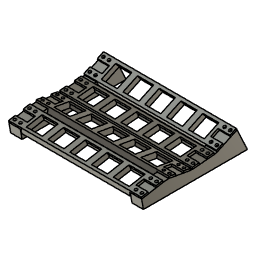
generator (Autodesk Fusion 360 design; units mm, degrees)
Autodesk Fusion 360 part; units mm, degrees
sketch "sketchRails" plane through (0, 0, 0) normal (1, 0, 0) x (0, 1, 0)
  line L0 (-1.7973, 10.1928) -> (16.9633, 13.5008)
  line L1 (22.5, 13.9365) -> (41.2606, 10.6285)
  line L2 (42.9622, 10.5542) -> (61.9397, 12.2146)
  line L3 (64.1312, 12.8018) -> (81.3964, 20.8527)
  line L4 (0, 0) -> (87.5485, 7.6595) construction
  line L5 (42.7693, 17.0622) -> (60.9996, 18.6571) construction
  line L6 (61.7241, 18.8513) -> (78.3095, 26.5852) construction
  line L7 (42.02, 17.0949) -> (23.998, 20.2727) construction
  line L8 (15.4653, 19.8369) -> (-2.5567, 16.6591) construction
  line L9 (78.3095, 26.5852) -> (72.1582, 32.3231) construction
  line L10 (72.1582, 32.3231) -> (61.2825, 27.2517) construction
  line L11 (61.2825, 27.2517) -> (61.7241, 18.8513) construction
  line L12 (60.9996, 18.6571) -> (57.1818, 26.1529) construction
  line L13 (57.1818, 26.1529) -> (45.2275, 25.1071) construction
  line L14 (45.2275, 25.1071) -> (42.7693, 17.0622) construction
  line L15 (42.02, 17.0949) -> (40.2723, 25.3234) construction
  line L16 (40.2723, 25.3234) -> (28.4546, 27.4072) construction
  line L17 (28.4546, 27.4072) -> (23.998, 20.2727) construction
  line L18 (15.4653, 19.8369) -> (11.0087, 26.9714) construction
  line L19 (11.0087, 26.9714) -> (-0.809, 24.8876) construction
  line L20 (-0.809, 24.8876) -> (-2.5567, 16.6591) construction
  line L21 (7.583, 11.8468) -> (6.4543, 18.248) construction
  line L22 (31.8803, 12.2825) -> (33.009, 18.6838) construction
  line L23 (52.451, 11.3844) -> (51.8844, 17.8597) construction
  line L24 (72.7638, 16.8272) -> (70.0168, 22.7182) construction
  line L25 (-1.7973, 10.1928) -> (16.9633, 13.5008)
  line L26 (16.9633, 13.5008) -> (17.2412, 11.9251)
  line L27 (17.2412, 11.9251) -> (-1.5194, 8.6171)
  line L28 (-1.5194, 8.6171) -> (-1.7973, 10.1928)
  line L29 (22.5, 13.9365) -> (41.2606, 10.6285)
  line L30 (41.2606, 10.6285) -> (40.9827, 9.0528)
  line L31 (40.9827, 9.0528) -> (22.2221, 12.3608)
  line L32 (22.2221, 12.3608) -> (22.5, 13.9365)
  line L33 (42.9622, 10.5542) -> (61.9397, 12.2146)
  line L34 (61.9397, 12.2146) -> (62.0792, 10.6206)
  line L35 (62.0792, 10.6206) -> (43.1016, 8.9603)
  line L36 (43.1016, 8.9603) -> (42.9622, 10.5542)
  line L37 (64.1312, 12.8018) -> (81.3964, 20.8527)
  line L38 (81.3964, 20.8527) -> (82.0726, 19.4026)
  line L39 (82.0726, 19.4026) -> (64.8074, 11.3517)
  line L40 (64.8074, 11.3517) -> (64.1312, 12.8018)
  line L41 (43.1016, 8.9603) -> (40.9827, 9.0528)
  line L42 (22.2221, 12.3608) -> (17.2412, 11.9251)
  line L43 (-1.5194, 8.6171) -> (0, 0)
  line L44 (42.7693, 17.0622) -> (42.02, 17.0949)
  line L45 (61.7241, 18.8513) -> (60.9996, 18.6571)
  line L46 (62.0792, 10.6206) -> (64.8074, 11.3517)
  line L47 (61.3618, 18.7542) -> (63.4433, 10.9862) construction
  line L48 (42.3946, 17.0786) -> (42.0422, 9.0066) construction
  line L49 (0, 0) -> (91.1201, 0)
  line L50 (91.1201, 0) -> (82.0726, 19.4026)
  dimension "d1" = 19.05
  dimension "d2" = 19.05
  dimension "d3" = 19.05
  dimension "d4" = 19.05
  dimension "d6" = 5
  dimension "d7" = 15
  dimension "d8" = 20
  dimension "d9" = 18.3
  dimension "d10" = 18.3
  dimension "d11" = 18.3
  dimension "d12" = 18.3
  dimension "d13" = 12
  dimension "d14" = 12
  dimension "d15" = 12
  dimension "d16" = 12
  dimension "d17" = 7.8
  dimension "d18" = 7.8
  dimension "d19" = 7.8
  dimension "d20" = 7.8
  dimension "d21" = 6.5
  dimension "d22" = 6.5
  dimension "d23" = 6.5
  dimension "d24" = 6.5
  dimension "d25" = 1.6
  dimension "d26" = 1.6
  dimension "d27" = 1.6
  dimension "d28" = 1.6
  dimension "d30" = 0.75
  dimension "d31" = 0.75
  dimension "d32" = 5
  dimension "d34" = 5
  dimension "d40" = 8.75
  dimension "validationClearance" = 8.9603
  constraint parallel L2 L4
  constraint parallel L2 L5
  constraint parallel L1 L7
  constraint parallel L0 L8
  constraint parallel L3 L6
  constraint parallel L6 L10
  constraint parallel L5 L13
  constraint parallel L7 L16
  constraint parallel L8 L19
  constraint equal L18 L20
  constraint equal L15 L17
  constraint equal L12 L14
  constraint equal L9 L11
  constraint midpoint L0 L21.start
  constraint midpoint L8 L21.end
  constraint midpoint L1 L22.start
  constraint midpoint L7 L22.end
  constraint midpoint L2 L23.start
  constraint midpoint L5 L23.end
  constraint midpoint L3 L24.start
  constraint midpoint L6 L24.end
  constraint perpendicular L3 L24
  constraint perpendicular L2 L23
  constraint perpendicular L1 L22
  constraint perpendicular L0 L21
  constraint perpendicular L25 L26
  constraint parallel L25 L27
  constraint parallel L26 L28
  constraint perpendicular L29 L30
  constraint parallel L29 L31
  constraint parallel L30 L32
  constraint perpendicular L33 L34
  constraint parallel L33 L35
  constraint parallel L34 L36
  constraint perpendicular L37 L38
  constraint parallel L37 L39
  constraint parallel L38 L40
  constraint coincident L4 L43.end
  constraint perpendicular L27 L43
  constraint midpoint L45 L47.start
  constraint midpoint L46 L47.end
  constraint midpoint L44 L48.start
  constraint midpoint L41 L48.end
  constraint perpendicular L41 L48
  constraint perpendicular L45 L47
  constraint perpendicular L44 L48
  constraint parallel L4 L42
  constraint horizontal L49
  constraint perpendicular L39 L50
  constraint coincident L4.start L43.end
  constraint coincident L4.end L50
  measures "d1" distance of L0.start L0.end
  measures "d2" distance of L1.start L1.end
  measures "d3" distance of L2.start L2.end
  measures "d4" distance of L3.start L3.end
  measures "d6" angle of L0 L4
  measures "d7" angle of L1 L4
  measures "d8" angle of L3 L4
  measures "d9" distance of L5.start L5.end
  measures "d10" distance of L6.start L6.end
  measures "d11" distance of L7.start L7.end
  measures "d12" distance of L8.start L8.end
  measures "d13" distance of L15.end L16.end
  measures "d14" distance of L18.end L19.end
  measures "d15" distance of L12.end L13.end
  measures "d16" distance of L9.end L10.end
  measures "d17" distance of L5 L13
  measures "d18" distance of L6 L10
  measures "d19" distance of L7 L16
  measures "d20" distance of L8 L19
  measures "d21" distance of L0 L8
  measures "d22" distance of L1 L7
  measures "d23" distance of L2 L5
  measures "d24" distance of L3 L6
  measures "d25" distance of L0.start L27.end
  measures "d26" distance of L1.start L31.end
  measures "d27" distance of L2.start L35.end
  measures "d28" distance of L3.start L39.end
  measures "d30" distance of L5.start L7.start
  measures "d31" distance of L5.end L6.start
  measures "d32" distance of L26.end L31.end
  measures "d34" angle of L4 L49
  measures "d40" distance of L27.end L4.start
  measures "validationClearance" distance of L35.end L49
extrude "extrudeRailLeft" add sketch "sketchRails" along normal blind 10 contours L27 L31 L35 L39 L41 L42 L43 L46 L49 L50 makes body 1
extrude "extrudeRailRight" add sketch "sketchRails" along normal blind 10 from surface at 106.3 separate body contours L27 L31 L35 L39 L41 L42 L43 L46 L49 L50 makes body 2
sketch "sketchPlateTop" plane through (0, 7.2271, -15.4985) normal (0, -0.422618, 0.906308) x (1, 0, 0)
  line L0 (0, 82.5829) -> (0, 63.5329)
  line L1 (0, 63.5329) -> (10, 63.5329)
  line L2 (10, 63.5329) -> (10, 82.5829)
  line L3 (10, 82.5829) -> (0, 82.5829)
  line L4 (106.3, 82.5829) -> (106.3, 63.5329)
  line L5 (106.3, 63.5329) -> (116.3, 63.5329)
  line L6 (116.3, 63.5329) -> (116.3, 82.5829)
  line L7 (116.3, 82.5829) -> (106.3, 82.5829)
  line L8 (0, 82.5829) -> (116.3, 82.5829)
  line L9 (116.3, 82.5829) -> (116.3, 63.5329)
  line L10 (116.3, 63.5329) -> (0, 63.5329)
  line L11 (0, 63.5329) -> (0, 82.5829)
  line L12 (0, 76.5829) -> (10.525, 76.5829)
  line L13 (10.525, 76.5829) -> (10.525, 69.5329)
  line L14 (10.525, 69.5329) -> (0, 69.5329)
  line L15 (0, 69.5329) -> (0, 76.5829)
  line L16 (116.3, 69.5329) -> (105.775, 69.5329)
  line L17 (105.775, 69.5329) -> (105.775, 76.5829)
  line L18 (105.775, 76.5829) -> (116.3, 76.5829)
  line L19 (116.3, 76.5829) -> (116.3, 69.5329)
  line L20 (13.05, 80.0579) -> (27.05, 80.0579)
  line L21 (27.05, 80.0579) -> (27.05, 66.0579)
  line L22 (27.05, 66.0579) -> (13.05, 66.0579)
  line L23 (13.05, 66.0579) -> (13.05, 80.0579)
  line L24 (32.1, 80.0579) -> (46.1, 80.0579)
  line L25 (46.1, 80.0579) -> (46.1, 66.0579)
  line L26 (46.1, 66.0579) -> (32.1, 66.0579)
  line L27 (32.1, 66.0579) -> (32.1, 80.0579)
  line L28 (51.15, 80.0579) -> (65.15, 80.0579)
  line L29 (65.15, 80.0579) -> (65.15, 66.0579)
  line L30 (65.15, 66.0579) -> (51.15, 66.0579)
  line L31 (51.15, 66.0579) -> (51.15, 80.0579)
  line L32 (70.2, 80.0579) -> (84.2, 80.0579)
  line L33 (84.2, 80.0579) -> (84.2, 66.0579)
  line L34 (84.2, 66.0579) -> (70.2, 66.0579)
  line L35 (70.2, 66.0579) -> (70.2, 80.0579)
  line L36 (89.25, 80.0579) -> (103.25, 80.0579)
  line L37 (103.25, 80.0579) -> (103.25, 66.0579)
  line L38 (103.25, 66.0579) -> (89.25, 66.0579)
  line L39 (89.25, 66.0579) -> (89.25, 80.0579)
  line L40 (5, 63.5329) -> (5, 69.5329) construction
  line L41 (5, 66.5329) -> (10, 66.5329) construction
  line L42 (5, 66.5329) -> (0, 66.5329) construction
  circle A0 centre (2.5, 66.5329) radius 1.5 construction
  circle A1 centre (7.5, 66.5329) radius 1.5 construction
  circle A2 centre (2.5, 66.5329) radius 1.2
  circle A3 centre (7.5, 66.5329) radius 1.2
  line L43 (0, 73.0579) -> (116.3, 73.0579) construction
  line L44 (58.15, 82.5829) -> (58.15, 63.5329) construction
  circle A4 centre (2.5, 79.5829) radius 1.2
  circle A5 centre (7.5, 79.5829) radius 1.2
  circle A6 centre (108.8, 79.5829) radius 1.2
  circle A7 centre (113.8, 79.5829) radius 1.2
  circle A8 centre (113.8, 66.5329) radius 1.2
  circle A9 centre (108.8, 66.5329) radius 1.2
  dimension "d47" = 10.525
  dimension "d48" = 7.05
  dimension "d49" = 10.525
  dimension "d50" = 7.05
  dimension "d51" = 6
  dimension "d52" = 6
  dimension "d53" = 14
  dimension "d54" = 14
  dimension "d55" = 2.525
  dimension "d56" = 2.525
  dimension "d59" = 19.05
  dimension "d60" = 0
  dimension "d138" = 3
  dimension "d139" = 3
  dimension "d140" = 2.4
  dimension "d141" = 2.4
  constraint horizontal L8
  constraint vertical L9
  constraint horizontal L10
  constraint vertical L11
  constraint coincident L5.end L6.start
  constraint coincident L0.start L3.end
  constraint horizontal L12
  constraint vertical L13
  constraint horizontal L14
  constraint vertical L15
  constraint coincident L0 L12.start
  constraint horizontal L16
  constraint vertical L17
  constraint horizontal L18
  constraint vertical L19
  constraint coincident L6 L16.start
  constraint horizontal L20
  constraint vertical L21
  constraint horizontal L22
  constraint vertical L23
  constraint midpoint L1 L40.start
  constraint coincident L14 L40.end
  constraint perpendicular L14 L40
  constraint midpoint L40 L41.start
  constraint coincident L2 L41.end
  constraint perpendicular L2 L41
  constraint coincident L11 L42.end
  constraint perpendicular L11 L42
  constraint midpoint L42 A0.centre
  constraint midpoint L41 A1.centre
  constraint concentric A0 A2
  constraint concentric A1 A3
  constraint midpoint L15 L43.start
  constraint midpoint L19 L43.end
  constraint midpoint L8 L44.start
  constraint midpoint L10 L44.end
  constraint symmetric A2 L43 A4
  constraint symmetric A3 L43 A5
  constraint symmetric A2 L44 A8
  constraint symmetric A3 L44 A9
  constraint symmetric L44 A4 A7
  constraint symmetric L44 A5 A6
  measures "d47" distance of L12.start L12.end
  measures "d48" distance of L12.start L14.end
  measures "d49" distance of L16.start L16.end
  measures "d50" distance of L16.start L18.end
  measures "d51" distance of L8 L12
  measures "d52" distance of L8 L18
  measures "d53" distance of L20.start L20.end
  measures "d54" distance of L20.start L22.end
  measures "d55" distance of L13 L23
  measures "d56" distance of L8 L20
  measures "d138" diameter of A0
  measures "d139" diameter of A1
  measures "d140" diameter of A2
  measures "d141" diameter of A3
hole "holeRailsTop" at (2.5, 79.3537, 18.1347) at (7.5, 79.3537, 18.1347) at (7.5, 67.5263, 12.6195) at (2.5, 67.5263, 12.6195) at (108.8, 79.3537, 18.1347) at (113.8, 79.3537, 18.1347) at (113.8, 67.5263, 12.6195) at (108.8, 67.5263, 12.6195) direction (0, 0.422618, -0.906308) diameter 1.8 depth 5 tip angle 180 bodies 1 2
extrude "extrudePlateTop" add sketch "sketchPlateTop" along normal blind 1.6 separate body contours L0 L2 L3 L8 L11 L12 | L2 L4 L8 L10 L12 L13 L14 L16 L17 L18 | L0 L1 L2 L10 L11 L14 | L4 L6 L7 L8 L9 L18 | L4 L5 L6 L9 L10 L16 makes body 3
sketch "sketchPlateMiddle" plane through (0, -0.4506, 5.15) normal (0, -0.087156, 0.996195) x (1, 0, 0)
  line L0 (0, 62.7686) -> (0, 43.7186)
  line L1 (0, 43.7186) -> (10, 43.7186)
  line L2 (10, 43.7186) -> (10, 62.7686)
  line L3 (10, 62.7686) -> (0, 62.7686)
  line L4 (106.3, 62.7686) -> (106.3, 43.7186)
  line L5 (106.3, 43.7186) -> (116.3, 43.7186)
  line L6 (116.3, 43.7186) -> (116.3, 62.7686)
  line L7 (116.3, 62.7686) -> (106.3, 62.7686)
  line L8 (0, 62.7686) -> (116.3, 62.7686)
  line L9 (116.3, 62.7686) -> (116.3, 43.7186)
  line L10 (116.3, 43.7186) -> (0, 43.7186)
  line L11 (0, 43.7186) -> (0, 62.7686)
  line L12 (0, 56.7686) -> (10.525, 56.7686)
  line L13 (10.525, 56.7686) -> (10.525, 49.7186)
  line L14 (10.525, 49.7186) -> (0, 49.7186)
  line L15 (0, 49.7186) -> (0, 56.7686)
  line L16 (116.3, 49.7186) -> (105.775, 49.7186)
  line L17 (105.775, 49.7186) -> (105.775, 56.7686)
  line L18 (105.775, 56.7686) -> (116.3, 56.7686)
  line L19 (116.3, 56.7686) -> (116.3, 49.7186)
  line L20 (13.05, 60.2436) -> (27.05, 60.2436)
  line L21 (27.05, 60.2436) -> (27.05, 46.2436)
  line L22 (27.05, 46.2436) -> (13.05, 46.2436)
  line L23 (13.05, 46.2436) -> (13.05, 60.2436)
  line L24 (32.1, 60.2436) -> (46.1, 60.2436)
  line L25 (46.1, 60.2436) -> (46.1, 46.2436)
  line L26 (46.1, 46.2436) -> (32.1, 46.2436)
  line L27 (32.1, 46.2436) -> (32.1, 60.2436)
  line L28 (51.15, 60.2436) -> (65.15, 60.2436)
  line L29 (65.15, 60.2436) -> (65.15, 46.2436)
  line L30 (65.15, 46.2436) -> (51.15, 46.2436)
  line L31 (51.15, 46.2436) -> (51.15, 60.2436)
  line L32 (70.2, 60.2436) -> (84.2, 60.2436)
  line L33 (84.2, 60.2436) -> (84.2, 46.2436)
  line L34 (84.2, 46.2436) -> (70.2, 46.2436)
  line L35 (70.2, 46.2436) -> (70.2, 60.2436)
  line L36 (89.25, 60.2436) -> (103.25, 60.2436)
  line L37 (103.25, 60.2436) -> (103.25, 46.2436)
  line L38 (103.25, 46.2436) -> (89.25, 46.2436)
  line L39 (89.25, 46.2436) -> (89.25, 60.2436)
  line L40 (5, 43.7186) -> (5, 49.7186) construction
  line L41 (5, 46.7186) -> (0, 46.7186) construction
  line L42 (5, 46.7186) -> (10, 46.7186) construction
  circle A0 centre (2.5, 46.7186) radius 1.2
  circle A1 centre (7.5, 46.7186) radius 1.2
  line L43 (0, 53.2436) -> (116.3, 53.2436) construction
  line L44 (58.15, 43.7186) -> (58.15, 62.7686) construction
  circle A2 centre (7.5, 59.7686) radius 1.2
  circle A3 centre (2.5, 59.7686) radius 1.2
  circle A4 centre (113.8, 46.7186) radius 1.2
  circle A5 centre (108.8, 46.7186) radius 1.2
  circle A6 centre (108.8, 59.7686) radius 1.2
  circle A7 centre (113.8, 59.7686) radius 1.2
  dimension "d63" = 10.525
  dimension "d64" = 7.05
  dimension "d65" = 10.525
  dimension "d66" = 7.05
  dimension "d67" = 6
  dimension "d68" = 6
  dimension "d69" = 14
  dimension "d70" = 14
  dimension "d71" = 2.525
  dimension "d72" = 2.525
  dimension "d75" = 19.05
  dimension "d76" = 0
  dimension "d142" = 2.4
  dimension "d143" = 2.4
  constraint horizontal L8
  constraint vertical L9
  constraint horizontal L10
  constraint vertical L11
  constraint coincident L5.end L6.start
  constraint coincident L0.start L3.end
  constraint horizontal L12
  constraint vertical L13
  constraint horizontal L14
  constraint vertical L15
  constraint coincident L0 L12.start
  constraint horizontal L16
  constraint vertical L17
  constraint horizontal L18
  constraint vertical L19
  constraint coincident L9 L16.start
  constraint horizontal L20
  constraint vertical L21
  constraint horizontal L22
  constraint vertical L23
  constraint midpoint L1 L40.start
  constraint coincident L14 L40.end
  constraint perpendicular L14 L40
  constraint midpoint L40 L41.start
  constraint coincident L0 L41.end
  constraint perpendicular L0 L41
  constraint coincident L2 L42.end
  constraint perpendicular L2 L42
  constraint midpoint L41 A0.centre
  constraint midpoint L42 A1.centre
  constraint midpoint L0 L43.start
  constraint midpoint L19 L43.end
  constraint midpoint L10 L44.start
  constraint midpoint L8 L44.end
  constraint symmetric A0 L43 A3
  constraint symmetric A1 L43 A2
  constraint symmetric A0 L44 A4
  constraint symmetric A1 L44 A5
  constraint symmetric L44 A2 A6
  constraint symmetric L44 A3 A7
  measures "d63" distance of L12.start L12.end
  measures "d64" distance of L12.start L14.end
  measures "d65" distance of L16.start L16.end
  measures "d66" distance of L16.start L18.end
  measures "d67" distance of L8 L18
  measures "d68" distance of L8 L12
  measures "d69" distance of L20.start L20.end
  measures "d70" distance of L20.start L22.end
  measures "d71" distance of L8 L20
  measures "d72" distance of L13 L23
  measures "d142" diameter of A0
  measures "d143" diameter of A1
hole "holeRailsMiddle" at (2.5, 59.0906, 10.3592) at (7.5, 46.0902, 9.2218) at (2.5, 46.0902, 9.2218) at (7.5, 59.0906, 10.3592) at (113.8, 46.0902, 9.2218) at (113.8, 59.0906, 10.3592) at (108.8, 46.0902, 9.2218) at (108.8, 59.0906, 10.3592) direction (0, 0.087156, -0.996195) diameter 1.8 depth 5 tip angle 180 bodies 1 2
extrude "extrudePlateMiddle" add sketch "sketchPlateMiddle" along normal blind 1.6 separate body contours L0 L2 L3 L8 L11 L12 | L2 L4 L8 L10 L12 L13 L14 L16 L17 L18 | L0 L1 L2 L10 L11 L14 | L4 L6 L7 L8 L9 L18 | L4 L5 L6 L9 L10 L16 makes body 4
sketch "sketchPlateBottom" plane through (0, 2.7839, 15.7883) normal (0, 0.173648, 0.984808) x (-1, 0, 0)
  line L0 (0, -38.7881) -> (0, -19.7381)
  line L1 (0, -19.7381) -> (-10, -19.7381)
  line L2 (-10, -19.7381) -> (-10, -38.7881)
  line L3 (-10, -38.7881) -> (0, -38.7881)
  line L4 (-106.3, -38.7881) -> (-106.3, -19.7381)
  line L5 (-106.3, -19.7381) -> (-116.3, -19.7381)
  line L6 (-116.3, -19.7381) -> (-116.3, -38.7881)
  line L7 (-116.3, -38.7881) -> (-106.3, -38.7881)
  line L8 (0, -38.7881) -> (-116.3, -38.7881)
  line L9 (-116.3, -38.7881) -> (-116.3, -19.7381)
  line L10 (-116.3, -19.7381) -> (0, -19.7381)
  line L11 (0, -19.7381) -> (0, -38.7881)
  line L12 (0, -32.7881) -> (-10.525, -32.7881)
  line L13 (-10.525, -32.7881) -> (-10.525, -25.7381)
  line L14 (-10.525, -25.7381) -> (0, -25.7381)
  line L15 (0, -25.7381) -> (0, -32.7881)
  line L16 (-116.3, -25.7381) -> (-105.775, -25.7381)
  line L17 (-105.775, -25.7381) -> (-105.775, -32.7881)
  line L18 (-105.775, -32.7881) -> (-116.3, -32.7881)
  line L19 (-116.3, -32.7881) -> (-116.3, -25.7381)
  line L20 (-13.05, -36.2631) -> (-27.05, -36.2631)
  line L21 (-27.05, -36.2631) -> (-27.05, -22.2631)
  line L22 (-27.05, -22.2631) -> (-13.05, -22.2631)
  line L23 (-13.05, -22.2631) -> (-13.05, -36.2631)
  line L24 (-32.1, -36.2631) -> (-46.1, -36.2631)
  line L25 (-46.1, -36.2631) -> (-46.1, -22.2631)
  line L26 (-46.1, -22.2631) -> (-32.1, -22.2631)
  line L27 (-32.1, -22.2631) -> (-32.1, -36.2631)
  line L28 (-51.15, -36.2631) -> (-65.15, -36.2631)
  line L29 (-65.15, -36.2631) -> (-65.15, -22.2631)
  line L30 (-65.15, -22.2631) -> (-51.15, -22.2631)
  line L31 (-51.15, -22.2631) -> (-51.15, -36.2631)
  line L32 (-70.2, -36.2631) -> (-84.2, -36.2631)
  line L33 (-84.2, -36.2631) -> (-84.2, -22.2631)
  line L34 (-84.2, -22.2631) -> (-70.2, -22.2631)
  line L35 (-70.2, -22.2631) -> (-70.2, -36.2631)
  line L36 (-89.25, -36.2631) -> (-103.25, -36.2631)
  line L37 (-103.25, -36.2631) -> (-103.25, -22.2631)
  line L38 (-103.25, -22.2631) -> (-89.25, -22.2631)
  line L39 (-89.25, -22.2631) -> (-89.25, -36.2631)
  line L40 (-111.3, -38.7881) -> (-111.0375, -32.7881) construction
  line L41 (-111.1688, -35.7881) -> (-116.3, -35.7881) construction
  line L42 (-111.1688, -35.7881) -> (-106.3, -35.7881) construction
  line L43 (0, -29.2631) -> (-116.3, -29.2631) construction
  line L44 (-58.15, -19.7381) -> (-58.15, -38.7881) construction
  circle A0 centre (-113.7344, -35.7881) radius 1.2
  circle A1 centre (-108.7344, -35.7881) radius 1.2
  circle A2 centre (-108.7344, -22.7381) radius 1.2
  circle A3 centre (-113.7344, -22.7381) radius 1.2
  circle A4 centre (-7.5656, -35.7881) radius 1.2
  circle A5 centre (-2.5656, -35.7881) radius 1.2
  circle A6 centre (-7.5656, -22.7381) radius 1.2
  circle A7 centre (-2.5656, -22.7381) radius 1.2
  dimension "d79" = 10.525
  dimension "d80" = 7.05
  dimension "d81" = 10.525
  dimension "d82" = 7.05
  dimension "d83" = 6
  dimension "d84" = 6
  dimension "d85" = 14
  dimension "d86" = 14
  dimension "d87" = 2.525
  dimension "d88" = 2.525
  dimension "d91" = 19.05
  dimension "d92" = 0
  dimension "d144" = 2.4
  dimension "d145" = 2.4
  constraint horizontal L8
  constraint vertical L9
  constraint horizontal L10
  constraint vertical L11
  constraint coincident L5.end L6.start
  constraint coincident L0.start L3.end
  constraint horizontal L12
  constraint vertical L13
  constraint horizontal L14
  constraint vertical L15
  constraint coincident L0 L12.start
  constraint horizontal L16
  constraint vertical L17
  constraint horizontal L18
  constraint vertical L19
  constraint coincident L6 L16.start
  constraint horizontal L20
  constraint vertical L21
  constraint horizontal L22
  constraint vertical L23
  constraint midpoint L7 L40.start
  constraint midpoint L18 L40.end
  constraint midpoint L40 L41.start
  constraint coincident L6 L41.end
  constraint perpendicular L6 L41
  constraint coincident L4 L42.end
  constraint perpendicular L4 L42
  constraint midpoint L11 L43.start
  constraint midpoint L19 L43.end
  constraint midpoint L10 L44.start
  constraint midpoint L8 L44.end
  constraint midpoint L41 A0.centre
  constraint midpoint L42 A1.centre
  constraint symmetric L43 A0 A3
  constraint symmetric L43 A1 A2
  constraint symmetric L44 A0 A5
  constraint symmetric L44 A1 A4
  constraint symmetric L44 A2 A6
  constraint symmetric L44 A3 A7
  measures "d79" distance of L12.start L12.end
  measures "d80" distance of L12.start L14.end
  measures "d81" distance of L16.start L16.end
  measures "d82" distance of L16.start L18.end
  measures "d83" distance of L8 L18
  measures "d84" distance of L8 L12
  measures "d85" distance of L20.start L20.end
  measures "d86" distance of L20.start L22.end
  measures "d87" distance of L8 L20
  measures "d88" distance of L13 L23
  measures "d144" diameter of A0
  measures "d145" diameter of A1
hole "holeRailsBottom" at (2.5656, 38.0283, 9.5738) at (7.5656, 38.0283, 9.5738) at (7.5656, 25.1766, 11.8399) at (2.5656, 25.1766, 11.8399) at (113.7344, 25.1766, 11.8399) at (113.7344, 38.0283, 9.5738) at (108.7344, 25.1766, 11.8399) at (108.7344, 38.0283, 9.5738) direction (0, -0.173648, -0.984808) diameter 1.8 depth 5 tip angle 180 bodies 1 2
extrude "extrudePlateBottom" add sketch "sketchPlateBottom" along normal blind 1.6 separate body contours L0 L2 L3 L8 L11 L12 | L2 L4 L8 L10 L12 L13 L14 L16 L17 L18 | L0 L1 L2 L10 L11 L14 | L4 L6 L7 L8 L9 L18 | L4 L5 L6 L9 L10 L16 makes body 5
sketch "sketchPlateThumb" plane through (0, -1.5194, 8.6171) normal (0, -0.173648, 0.984808) x (1, 0, 0)
  line L0 (0, 19.05) -> (0, 0)
  line L1 (0, 0) -> (10, 0)
  line L2 (10, 0) -> (10, 19.05)
  line L3 (10, 19.05) -> (0, 19.05)
  line L4 (106.3, 19.05) -> (106.3, 0)
  line L5 (106.3, 0) -> (116.3, 0)
  line L6 (116.3, 0) -> (116.3, 19.05)
  line L7 (116.3, 19.05) -> (106.3, 19.05)
  line L8 (0, 19.05) -> (116.3, 19.05)
  line L9 (116.3, 19.05) -> (116.3, 0)
  line L10 (116.3, 0) -> (0, 0)
  line L11 (0, 0) -> (0, 19.05)
  line L12 (0, 13.05) -> (10.525, 13.05)
  line L13 (10.525, 13.05) -> (10.525, 6)
  line L14 (10.525, 6) -> (0, 6)
  line L15 (0, 6) -> (0, 13.05)
  line L16 (116.3, 6) -> (105.775, 6)
  line L17 (105.775, 6) -> (105.775, 13.05)
  line L18 (105.775, 13.05) -> (116.3, 13.05)
  line L19 (116.3, 13.05) -> (116.3, 6)
  line L20 (13.05, 16.525) -> (27.05, 16.525)
  line L21 (27.05, 16.525) -> (27.05, 2.525)
  line L22 (27.05, 2.525) -> (13.05, 2.525)
  line L23 (13.05, 2.525) -> (13.05, 16.525)
  line L24 (32.1, 16.525) -> (46.1, 16.525)
  line L25 (46.1, 16.525) -> (46.1, 2.525)
  line L26 (46.1, 2.525) -> (32.1, 2.525)
  line L27 (32.1, 2.525) -> (32.1, 16.525)
  line L28 (51.15, 16.525) -> (65.15, 16.525)
  line L29 (65.15, 16.525) -> (65.15, 2.525)
  line L30 (65.15, 2.525) -> (51.15, 2.525)
  line L31 (51.15, 2.525) -> (51.15, 16.525)
  line L32 (70.2, 16.525) -> (84.2, 16.525)
  line L33 (84.2, 16.525) -> (84.2, 2.525)
  line L34 (84.2, 2.525) -> (70.2, 2.525)
  line L35 (70.2, 2.525) -> (70.2, 16.525)
  line L36 (89.25, 16.525) -> (103.25, 16.525)
  line L37 (103.25, 16.525) -> (103.25, 2.525)
  line L38 (103.25, 2.525) -> (89.25, 2.525)
  line L39 (89.25, 2.525) -> (89.25, 16.525)
  line L40 (111.3, 19.05) -> (111.3, 13.05) construction
  line L41 (111.3, 16.05) -> (116.3, 16.05) construction
  line L42 (111.3, 16.05) -> (106.3, 16.05) construction
  line L43 (58.15, 19.05) -> (58.15, 0) construction
  line L44 (116.3, 9.525) -> (0, 9.525) construction
  circle A0 centre (113.8, 16.05) radius 1.2
  circle A1 centre (108.8, 16.05) radius 1.2
  circle A2 centre (113.8, 3) radius 1.2
  circle A3 centre (108.8, 3) radius 1.2
  circle A4 centre (7.5, 16.05) radius 1.2
  circle A5 centre (2.5, 16.05) radius 1.2
  circle A6 centre (7.5, 3) radius 1.2
  circle A7 centre (2.5, 3) radius 1.2
  dimension "d95" = 10.525
  dimension "d96" = 7.05
  dimension "d97" = 10.525
  dimension "d98" = 7.05
  dimension "d99" = 6
  dimension "d100" = 6
  dimension "d101" = 14
  dimension "d102" = 14
  dimension "d103" = 2.525
  dimension "d104" = 2.525
  dimension "d107" = 19.05
  dimension "d108" = 0
  dimension "d146" = 2.4
  dimension "d147" = 2.4
  constraint horizontal L8
  constraint vertical L9
  constraint horizontal L10
  constraint vertical L11
  constraint coincident L5.end L6.start
  constraint coincident L0.start L3.end
  constraint horizontal L12
  constraint vertical L13
  constraint horizontal L14
  constraint vertical L15
  constraint coincident L0 L12.start
  constraint horizontal L16
  constraint vertical L17
  constraint horizontal L18
  constraint vertical L19
  constraint coincident L9 L16.start
  constraint horizontal L20
  constraint vertical L21
  constraint horizontal L22
  constraint vertical L23
  constraint midpoint L7 L40.start
  constraint coincident L18 L40.end
  constraint perpendicular L18 L40
  constraint midpoint L40 L41.start
  constraint coincident L9 L41.end
  constraint perpendicular L9 L41
  constraint coincident L4 L42.end
  constraint perpendicular L4 L42
  constraint midpoint L8 L43.start
  constraint midpoint L10 L43.end
  constraint midpoint L9 L44.start
  constraint midpoint L15 L44.end
  constraint midpoint L41 A0.centre
  constraint midpoint L42 A1.centre
  constraint symmetric L44 A0 A2
  constraint symmetric L44 A1 A3
  constraint symmetric L43 A0 A5
  constraint symmetric L43 A1 A4
  constraint symmetric L43 A2 A7
  constraint symmetric L43 A3 A6
  measures "d95" distance of L12.start L12.end
  measures "d96" distance of L12.start L14.end
  measures "d97" distance of L16.start L16.end
  measures "d98" distance of L16.start L18.end
  measures "d99" distance of L8 L18
  measures "d100" distance of L8 L12
  measures "d101" distance of L20.start L20.end
  measures "d102" distance of L20.start L22.end
  measures "d103" distance of L8 L20
  measures "d104" distance of L13 L23
  measures "d146" diameter of A0
  measures "d147" diameter of A1
hole "holeRailsThumb" at (2.5, 14.2867, 11.4041) at (7.5, 14.2867, 11.4041) at (7.5, 1.435, 9.138) at (2.5, 1.435, 9.138) at (113.8, 1.435, 9.138) at (108.8, 1.435, 9.138) at (113.8, 14.2867, 11.4041) at (108.8, 14.2867, 11.4041) direction (0, 0.173648, -0.984808) diameter 1.8 depth 5 tip angle 180 bodies 1 2
extrude "extrudePlateThumb" add sketch "sketchPlateThumb" along normal blind 1.6 separate body contours L0 L2 L3 L8 L11 L12 | L2 L4 L8 L10 L12 L13 L14 L16 L17 L18 | L0 L1 L2 L10 L11 L14 | L4 L6 L7 L8 L9 L18 | L4 L5 L6 L9 L10 L16 makes body 6
sketch "sketchBumponCutout" plane through (0, 0, 0) normal (0, 0, -1) x (1, 0, 0)
  line L0 (106.3, -91.1201) -> (116.3, -91.1201)
  line L1 (0, -91.1201) -> (10, -91.1201)
  line L2 (0, 0) -> (10, 0)
  line L3 (106.3, 0) -> (116.3, 0)
  line L4 (111.3, -91.1201) -> (111.3, 0)
  line L5 (5, -91.1201) -> (5, 0)
  point P0 (5, -86.1201)
  point P1 (111.3, -86.1201)
  point P2 (111.3, -5)
  point P3 (5, -5)
  dimension "d156" = 5
  dimension "d157" = 5
  dimension "d158" = 5
  dimension "d159" = 5
  constraint midpoint L0 L4.start
  constraint midpoint L3 L4.end
  constraint midpoint L1 L5.start
  constraint midpoint L2 L5.end
  constraint coincident L5 P0
  constraint coincident L4 P1
  constraint coincident L4 P2
  constraint coincident L5 P3
  measures "d156" distance of L2 P3
  measures "d157" distance of L1 P0
  measures "d158" distance of L0 P1
  measures "d159" distance of L3 P2
hole "holeBumponCutout" at (5, 5, 0) at (111.3, 5, 0) at (5, 86.1201, 0) at (111.3, 86.1201, 0) direction (0, 0, 1) diameter 6.2 depth 0.6 tip angle 180 bodies 1 2
sketch "sketchRailsCutout" plane through (116.3, 0, 0) normal (1, 0, 0) x (0, 1, 0)
  line L0 (62.0792, 10.6206) -> (43.1016, 8.9603)
  line L1 (43.1016, 8.9603) -> (40.9827, 9.0528)
  line L2 (40.9827, 9.0528) -> (22.2221, 12.3608)
  line L3 (22.2221, 12.3608) -> (17.2412, 11.9251)
  line L4 (17.2412, 11.9251) -> (-1.5194, 8.6171)
  line L5 (-1.5194, 8.6171) -> (0, 0)
  line L6 (0, 0) -> (91.1201, 0)
  line L7 (91.1201, 0) -> (82.0726, 19.4026)
  line L8 (82.0726, 19.4026) -> (64.8074, 11.3517)
  line L9 (64.8074, 11.3517) -> (62.0792, 10.6206)
  line L10 (74.1424, 15.7047) -> (81.4656, 0)
  line L11 (7.0976, 10.1365) -> (8.885, 0)
  line L12 (20.0783, 4.1427) -> (19.7317, 12.143) construction
  line L13 (41.6932, 1.0142) -> (42.0422, 9.0066) construction
  line L14 (65.5138, 3.2588) -> (63.4433, 10.9862) construction
  circle A0 centre (19.9396, 7.3428) radius 1.2
  circle A1 centre (41.8328, 4.2112) radius 1.2
  circle A2 centre (64.6856, 6.3497) radius 1.2
  line L15 (85.4535, 12.1521) -> (67.554, 3.8054)
  line L16 (67.554, 3.8054) -> (63.4737, 2.7121)
  line L17 (63.4737, 2.7121) -> (43.2765, 0.9451)
  line L18 (43.2765, 0.9451) -> (40.1099, 1.0833)
  line L19 (40.1099, 1.0833) -> (21.8702, 4.2995)
  line L20 (21.8702, 4.2995) -> (18.2864, 3.986)
  line L21 (18.2864, 3.986) -> (-0.1302, 0.7386)
  dimension "d130" = -8
  dimension "d131" = 8.75
  dimension "d132" = 8.75
  dimension "d148" = 2.4
  dimension "d149" = 2.4
  dimension "d150" = 2.4
  dimension "d151" = 3.2
  dimension "d152" = 3.2
  dimension "validationAngle" = 65
  dimension "d185" = 3.2
  constraint coincident L8 L10.start
  constraint coincident L6 L10.end
  constraint perpendicular L8 L10
  constraint coincident L4 L11.start
  constraint coincident L6 L11.end
  constraint perpendicular L11 L21
  constraint midpoint L3 L12.end
  constraint midpoint L13.start L18
  constraint midpoint L1 L13.end
  constraint midpoint L14.start L16
  constraint midpoint L9 L14.end
  constraint coincident L12 A0.centre
  constraint coincident L13 A1.centre
  constraint coincident L14 A2.centre
  constraint coincident L12.start L20
  constraint midpoint L12.start L20
  measures "d131" distance of L5 L11
  measures "d132" distance of L7 L10
  measures "d148" diameter of A0
  measures "d149" diameter of A1
  measures "d150" diameter of A2
  measures "d151" distance of A2.centre L16
  measures "d152" distance of A1.centre L18
  measures "validationAngle" angle of L6 L7
  measures "d185" distance of A0.centre L20
extrude "extrudeRailsCutout" [suppressed]
extrude "extrudeThiccTop" add sketch "sketchPlateTop" against normal blind 3.4 separate body contours L2 L4 L8 L10 L12 L13 L14 L16 L17 L18 makes body 7
extrude "extrudeThiccMiddle" add sketch "sketchPlateMiddle" against normal blind 3.4 separate body contours L2 L4 L8 L10 L12 L13 L14 L16 L17 L18 makes body 8
extrude "extrudeThiccBottom" add sketch "sketchPlateBottom" against normal blind 3.4 separate body contours L2 L4 L8 L10 L12 L13 L14 L16 L17 L18 makes body 9
extrude "extrudeThiccThumb" add sketch "sketchPlateThumb" against normal blind 3.4 separate body contours L2 L4 L8 L10 L12 L13 L14 L16 L17 L18 makes body 10
move_face "cutoutThiccSides" offset -0.525 16 faces at (10, 36.8467, 8.6313) (10, 25.7678, 9.434) (106.3, 38.8163, 8.284) (106.3, 23.7982, 9.7813) (10, 81.2179, 16.503) (10, 69.3906, 10.9879) (106.3, 78.9263, 16.6849) (106.3, 69.3906, 10.9879) (10, 15.6652, 9.3455) (10, 0.647, 7.8482) (106.3, 15.6652, 9.3455) (106.3, 2.6166, 8.1955) (10, 58.2919, 8.014) (10, 47.1852, 8.1799) (106.3, 60.1855, 9.3173) (106.3, 45.2916, 6.8766) on bodies 7 8 9 10
move_face "cutoutSwitchClips" offset -0.8 40 faces at (22.3833, 38.1025, 7.2591) (36.7667, 38.2993, 8.3752) (55.8167, 38.2993, 8.3752) (74.8667, 38.2993, 8.3752) (93.9167, 38.2993, 8.3752) (93.9167, 24.3152, 9.6902) (74.8667, 24.3152, 9.6902) (60.4833, 24.512, 10.8063) (41.4333, 24.3152, 9.6902) (17.7167, 24.3152, 9.6902) (22.3833, 80.7421, 16.2812) (36.7667, 80.2631, 17.3083) (55.8167, 80.2631, 17.3083) (74.8667, 80.2631, 17.3083) (98.5833, 80.7421, 16.2812) (93.9167, 68.0538, 10.3645) (74.8667, 68.0538, 10.3645) (60.4833, 67.5748, 11.3916) (36.7667, 67.5748, 11.3916) (17.7167, 67.5748, 11.3916) (93.9167, 14.9513, 10.3705) (17.7167, 14.9513, 10.3705) (36.7667, 14.9513, 10.3705) (55.8167, 14.9513, 10.3705) (74.8667, 14.9513, 10.3705) (17.7167, 1.3608, 6.8233) (36.7667, 1.3608, 6.8233) (93.9167, 1.3608, 6.8233) (74.8667, 1.3608, 6.8233) (55.8167, 1.3608, 6.8233) (93.9167, 59.7613, 8.1425) (74.8667, 59.6625, 9.2716) (22.3833, 59.7613, 8.1425) (36.7667, 59.6625, 9.2716) (55.8167, 59.6625, 9.2716) (98.5833, 45.8146, 6.9224) (79.5333, 45.7158, 8.0514) (60.4833, 45.8146, 6.9224) (41.4333, 45.8146, 6.9224) (22.3833, 45.7158, 8.0514) on bodies 7 8 9 10
combine "combineThiccPlateTop" operation add target body 3 tool bodies 7
combine "combineThiccPlateMiddle" operation add target body 8 tool bodies 4
combine "combineThiccPlateBottom" operation add target body 9 tool bodies 5
combine "combineThiccPlateThumb" operation add target body 10 tool bodies 6
equation "d6 = plateThumbAngle"
equation "d7 = plateBottomAngle"
equation "d8 = plateTopAngle"
equation "d32 = plateThumbOffset"
equation "d34 = plateMiddleAngle"
equation "plateTopAngle = 20 deg" comment "relative to middle row"
equation "plateBottomAngle = 15 deg" comment "relative to middle row"
equation "plateThumbAngle = 5 deg" comment "relative to middle row"
equation "plateThumbOffset = 5 mm" comment ">0; prevent switch interference with bottom row"
equation "plateMiddleAngle = 5 deg" comment "relative to horizontal"
equation "validationClearance = 8.96033242 mm" comment ">=8mm probably"
equation "d44 = ( 19.05 * 5 ) * 1 mm + 11.05 mm"
equation "d152 = d151"
equation "validationAngle = 65.00 deg" comment ">=45deg for ease of printing"
equation "d161 = railHoleDepth"
equation "d162 = railHoleDiameter"
equation "d164 = railHoleDepth"
equation "d165 = railHoleDiameter"
equation "d167 = railHoleDepth"
equation "d168 = railHoleDiameter"
equation "d170 = railHoleDepth"
equation "d171 = railHoleDiameter"
equation "railHoleDepth = 5 mm" comment "ok for 6mm self tap or heat set insert"
equation "railHoleDiameter = 1.8 mm" comment "1.8mm m2 self tap; 3.4mm heat set insert"
equation "d185 = d151"
named bodies: "railLeft", "railRight", "plateTop", "plateMiddle", "plateBottom", "plateThumb"
